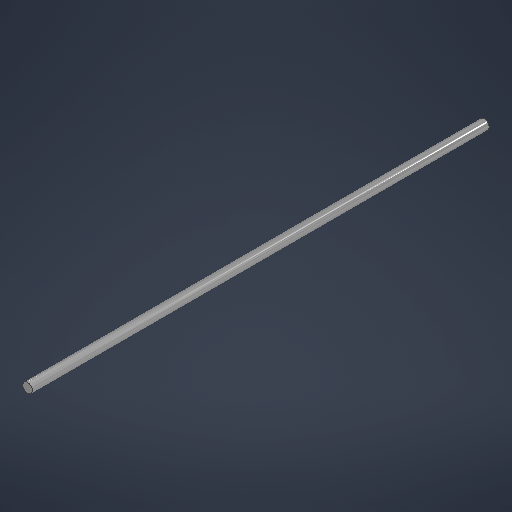
# Autodesk Inventor part: Threaded Rod
Saved by Autodesk Inventor 2026.1 (Build 301233020, 233B)
## iProperties
Created: 2026-04-07
Part Number: Threaded Rod
Material: Generic
Document SubType Name: Modeling
Designer: Bahaa
Mass: 0.589049 g
Surface Area: 9.52295 cm^2
Volume: 0.589049 cm^3
Density: 1 g/cm^3
Appearance: Default
Author: Bahaa
Autodesk Inventor part; units mm, degrees
ref_plane "YZ Plane" through (0, 0, 0) normal (1, 0, 0) x (0, 1, 0)
ref_plane "XZ Plane" through (0, 0, 0) normal (0, 1, 0) x (-1, 0, 0)
ref_plane "XY Plane" through (0, 0, 0) normal (0, 0, 1) x (1, 0, 0)
sketch "Sketch1" plane through (0, 0, 0) normal (0, 1, 0) x (-1, 0, 0)
  circle A0 centre (0, 0) radius 1.25
  dimension "d0" = 2.5
  constraints: 1 centre point, 1 coincident
  measures "d0" diameter of A0
extrude "Extrusion1" add sketch "Sketch1" along normal blind 120
body "Solid1"
